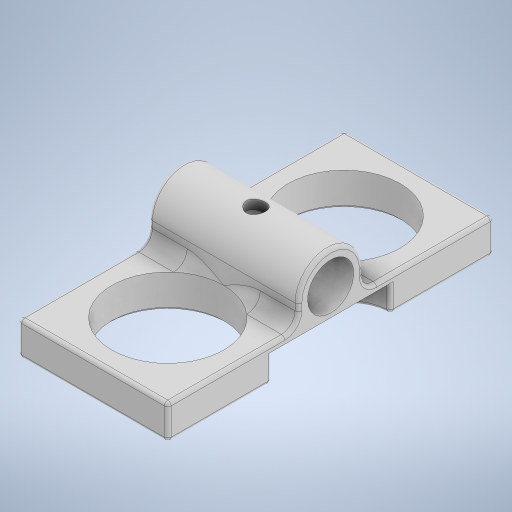
# Autodesk Inventor part: v2sensormount
Saved by Autodesk Inventor 2024.2 (Build 282272000, 272)
## iProperties
Created: 2024-01-15
Part Number: v2sensormount
Material: Generic
Document SubType Name: Modeling
Designer: Eric
Density: 1 g/cm^3
Appearance: Default
Author: Eric
Autodesk Inventor part; units mm, degrees
ref_plane "YZ Plane" through (0, 0, 0) normal (1, 0, 0) x (0, 1, 0)
ref_plane "XZ Plane" through (0, 0, 0) normal (0, 1, 0) x (-1, 0, 0)
sketch "Sketch1" plane through (0, 0, 0) normal (0, 1, 0) x (-1, 0, 0)
  circle A0 centre (0, 13) radius 8.25
  circle A1 centre (0, -13) radius 8.25
  line L0 (11, -24) -> (-11, -24)
  line L1 (-11, -24) -> (-11, 24)
  line L2 (-11, 24) -> (11, 24)
  line L3 (11, 24) -> (11, -24)
  point P0 (0, 0)
  dimension "d0" = 16.5
  dimension "d1" = 26
  dimension "d2" = 13
  dimension "d3" = 11
  dimension "d4" = 11
  dimension "d5" = 11
  dimension "d6" = 11
  constraints: 8 end point, 2 centre point, 2 parallel, 2 vertical alignment, 1 equal radius, 1 horizontal, 1 perpendicular
  measures "d0" diameter of A1
  measures "d1" distance of A0.centre A1.centre
  measures "d2" distance of point (0, 0) A1.centre
  measures "d3" distance from line of L0 A1.centre
  measures "d4" distance from line of L2 A0.centre
  measures "d5" distance from line of L3 A1.centre
  measures "d6" distance from line of L1 A1.centre
extrude "Extrusion1" add sketch "Sketch1" along normal blind 5
sketch "Sketch2" plane through (11, 0, 24) normal (1, 0, 0) x (0, 0, -1)
  circle A0 centre (24, 8) radius 3.4
  circle A1 centre (24, 8) radius 4.75
  line L0 (0, 0) -> (48, 0) projected
  line L1 (2.75, 5) -> (19.25, 5) projected
  line L2 (19.25, 5) -> (19.25, 8)
  line L3 (28.75, 5) -> (45.25, 5) projected
  line L4 (28.75, 8) -> (28.75, 5)
  line L5 (0, 5) -> (48, 5) projected
  point P0 (24, 0)
  point P1 (24, 0)
  point P2 (25.6, 5)
  point P3 (22.4, 5)
  point P4 (27.6827, 5)
  point P5 (20.3173, 5)
  dimension "d10" = 9.5
  dimension "d9" = 6.8
  dimension "d11" = 8
  constraints: 4 end point, 3 vertical, 1 centre point, 1 coincident, 1 midpoint, 3 other
  measures "d9" diameter of A0
  measures "d11" distance from line of L0 A0.centre
extrude "Extrusion2" add sketch "Sketch2" against normal up to surface (22 mm away) contours A0 L5 A1 | L5 L2 A1 | A1 L4 L5 picked at (28.254, 8.3789)
extrude "Extrusion3" cut sketch "Sketch2" against normal through all contours L5 A0 picked at (24.2749, 4.9005)
sketch "Sketch3" plane through (0, 0, 0) normal (0, -1, 0) x (1, 0, 0)
  line L0 (11, 2.5) -> (11, -2.5) construction
  line L1 (4.75, 2.5) -> (4.75, -2.5)
  line L2 (17.25, -2.5) -> (17.25, 2.5)
  arc A0 (17.25, 2.5) -> (4.75, 2.5) centre (11, 2.5) ccw
  arc A1 (4.75, -2.5) -> (17.25, -2.5) centre (11, -2.5) ccw
  line L3 (11, 24) -> (11, -24) projected
  line L4 (-11, 24) -> (11, 24) projected
  line L5 (0, 24) -> (0, -24) construction
  line L6 (-11, 2.5) -> (-11, -2.5) construction
  line L7 (-4.75, 2.5) -> (-4.75, -2.5)
  line L8 (-17.25, -2.5) -> (-17.25, 2.5)
  arc A2 (-4.75, 2.5) -> (-17.25, 2.5) centre (-11, 2.5) ccw
  arc A3 (-17.25, -2.5) -> (-4.75, -2.5) centre (-11, -2.5) ccw
  point P0 (0, 0)
  point P1 (11, 0)
  point P2 (-11, 0)
  dimension "d18" = 12.5
  dimension "d19" = 5
  constraints: 18 end point, 8 point on circle, 7 symmetric about line, 4 centre point, 4 tangent, 2 midpoint, 2 vertical, 1 collinear, 1 horizontal alignment, 1 parallel, 2 other
  measures "d18" distance between parallel lines of L2 L1
  measures "d19" distance of L0.start L0.end
extrude "Extrusion4" cut sketch "Sketch3" against normal blind 4
fillet "Fillet1" radius 2 4 edges at (-5.5, 5, -4.75) (5.5, 5, -4.75) (5.5, 5, 4.75) (-5.5, 5, 4.75)
fillet "Fillet2" radius 0.5 8 edges at (-11, 2.5, -24) (11, 2.5, -24) (-11, 2.5, 24) (11, 2.5, 24) (-11, 2, 8.75) (-11, 2, -8.75) (11, 2, -8.75) (11, 2, 8.75)
fillet "Fillet3" radius 0.5 40 edges at (-10.8536, 5, 23.8536) (0, 5, 24) (10.8536, 5, 23.8536) (11, 5, 15.125) (11, 5.5858, 5.3358) (11, 7.5, 4.75) (11, 12.75, 0) (11, 7.5, -4.75) (11, 5.5858, -5.3358) (11, 5, -15.125) (10.8536, 5, -23.8536) (0, 5, -24) (-10.8536, 5, -23.8536) (-11, 5, -15.125) (-11, 5.5858, -5.3358) (-11, 7.5, -4.75) (-11, 12.75, 0) (-11, 7.5, 4.75) (-11, 5.5858, 5.3358) (-11, 5, 15.125) (-10.8536, 0, 23.8536) (0, 0, 24) (10.8536, 0, 23.8536) (11, 0, 16.3657) (10.8664, 0, 8.8912) (6.4198, 0, 6.7526) (4.75, 0, 0) (6.4198, 0, -6.7526) (10.8664, 0, -8.8912) (11, 0, -16.3657) (10.8536, 0, -23.8536) (0, 0, -24) (-10.8536, 0, -23.8536) (-11, 0, -16.3657) (-10.8664, 0, -8.8912) (-6.4198, 0, -6.7526) (-4.75, 0, 0) (-6.4198, 0, 6.7526) (-10.8664, 0, 8.8912) (-11, 0, 16.3657)
chamfer "Chamfer1" distance 0.5 angle 45 2 edges at (8.25, 0, 13) (8.25, 0, -13)
ref_plane "Work Plane1" through (0, 15, 0) normal (0, 1, 0) x (1, 0, 0)
sketch "Sketch4" plane through (0, 15, 0) normal (0, 1, 0) x (1, 0, 0)
  circle A0 centre (0, 0) radius 1.4
  line L0 (11, 3.4) -> (11, -3.4) projected
  point P0 (0, 0)
  point P1 (11, 0)
  dimension "d29" = 2.8
  constraints: 1 centre point, 1 coincident, 1 horizontal alignment, 1 midpoint
  measures "d29" diameter of A0
extrude "Extrusion5" cut sketch "Sketch4" against normal up to surface round surface about axis through (11, 8, 0) along (-1, 0, 0) radius 3.4 far side no
body "Solid1"
